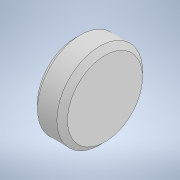
# Autodesk Inventor part: 711112
Saved by Autodesk Inventor 2022 (Build 260153000, 153)
## iProperties
Created: 2021-10-21
Part Number: 711112
Material: Типовые
Document SubType Name: Modeling
Designer: RaNSiD
Density: 1 g/cm^3
Appearance: По умолчанию
Author: RaNSiD
Autodesk Inventor part; units mm, degrees
ref_plane "YZ Plane" through (0, 0, 0) normal (1, 0, 0) x (0, 1, 0)
ref_plane "XZ Plane" through (0, 0, 0) normal (0, 1, 0) x (-1, 0, 0)
ref_plane "XY Plane" through (0, 0, 0) normal (0, 0, 1) x (1, 0, 0)
sketch "Эскиз1" plane through (0, 0, 0) normal (0, 0, 1) x (1, 0, 0)
  line L0 (0, 0) -> (20, 0)
  line L1 (0, 0) -> (0, 25)
  line L2 (0, 25) -> (3.5355, 28.5355)
  line L3 (20, 0) -> (20, 25)
  line L4 (20, 25) -> (16.4645, 28.5355)
  line L5 (16.4645, 28.5355) -> (3.5355, 28.5355)
  dimension "d0" = 20
  dimension "d1" = 25
  dimension "d2" = 5
  dimension "d3" = 135
  dimension "d4" = 5
  dimension "d5" = 135
  constraints: 12 end point, 2 vertical, 1 horizontal, 1 perpendicular
  measures "d0" distance of L0.start L0.end
  measures "d1" distance of L0.start L1.end
  measures "d2" distance of L1.end L2.end
  measures "d3" angle of L1 L2
  measures "d4" distance of L3.end L4.end
  measures "d5" angle of L3 L4
revolve "Вращение1" add sketch "Эскиз1" angle 360 about axis through (0, 0, 0) along (1, 0, 0)
sketch "Эскиз2" plane through (0, 0, 0) normal (-1, 0, 0) x (0, 0, 1)
  line L0 (0, 0) -> (0, 10) construction
  dimension "d7" = 10
  constraints: 2 end point, 1 coincident, 1 vertical
  measures "d7" distance of L0.start L0.end
hole "Отверстие1" at (0, 10, 0) direction (1, 0, 0) diameter 10 depth 8 tip angle 118 countersink diameter 15 countersink angle 90
